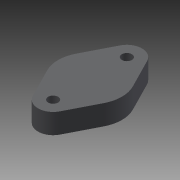
# Autodesk Inventor part: shaftPlug22
Saved by Autodesk Inventor 2013 (Build 170138000, 138)
## iProperties
Created: 2015-01-14
Part Number: shaftPlug22
Material: Generic
Document SubType Name: Modeling
Designer: dzban
Density: 1 g/cm^3
Author: dzban
Autodesk Inventor part; units mm, degrees
ref_plane "YZ Plane" through (0, 0, 0) normal (1, 0, 0) x (0, 1, 0)
ref_plane "XZ Plane" through (0, 0, 0) normal (0, 1, 0) x (-1, 0, 0)
ref_plane "XY Plane" through (0, 0, 0) normal (0, 0, 1) x (1, 0, 0)
sketch "Sketch1" plane through (0, 0, 0) normal (0, 0, 1) x (1, 0, 0)
  line L0 (-8.4619, -4.3182) -> (-4.0083, -13.0455)
  arc A0 (-4.0083, -13.0455) -> (4.0083, -13.0455) centre (0, -11) ccw
  line L1 (4.0083, -13.0455) -> (8.4619, -4.3182)
  arc A1 (8.4619, -4.3182) -> (8.4619, 4.3182) centre (0, 0) ccw
  line L2 (8.4619, 4.3182) -> (4.0083, 13.0455)
  arc A2 (4.0083, 13.0455) -> (-4.0083, 13.0455) centre (0, 11) ccw
  line L3 (-4.0083, 13.0455) -> (-8.4619, 4.3182)
  arc A3 (-8.4619, 4.3182) -> (-8.4619, -4.3182) centre (0, 0) ccw
  circle A4 centre (0, 11) radius 1.5
  circle A5 centre (0, -11) radius 1.5
  point P0 (0, 0)
  constraints: 8 end point, 8 point on circle, 6 centre point
extrude "Extrusion1" add sketch "Sketch1" along normal blind 6
body "Solid1"
